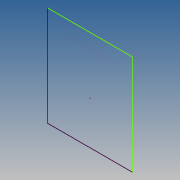
# Autodesk Inventor part: MountingBracket
Saved by Autodesk Inventor 2019 (Build 230136000, 136)
## iProperties
Created: 2019-12-19
Part Number: MountingBracket
Material: Generic
Document SubType Name: Modeling
Designer: voigt
Density: 1 g/cm^3
Appearance: Default
Author: voigt
Autodesk Inventor part; units mm, degrees
ref_plane "YZ Plane" through (0, 0, 0) normal (1, 0, 0) x (0, 1, 0)
ref_plane "XZ Plane" through (0, 0, 0) normal (0, 1, 0) x (-1, 0, 0)
ref_plane "XY Plane" through (0, 0, 0) normal (0, 0, 1) x (1, 0, 0)
sketch "Sketch1" plane through (0, 0, 0) normal (0, 0, 1) x (1, 0, 0)
  line L0 (20.828, 60.2998) -> (-20.828, 60.2998) construction
  line L1 (-38.1, 60.2998) -> (-38.1, 136.4998) construction
  line L2 (-38.1, 136.4998) -> (-20.828, 136.4998) construction
  line L3 (38.1, 136.4998) -> (-38.1, 136.4998) construction
  line L4 (37.846, 60.2998) -> (37.846, 136.4998) construction
  line L5 (-20.828, 47.6808) -> (-38.1, 47.6808) construction
  line L6 (-38.1, 136.4998) -> (37.846, 136.4998)
  line L7 (37.846, 136.4998) -> (37.846, 225.3188)
  line L8 (37.846, 225.3188) -> (-38.1, 225.3188)
  line L9 (-38.1, 225.3188) -> (-38.1, 136.4998)
  point P0 (0, 0)
  constraints: 8 end point, 2 parallel, 1 horizontal, 1 perpendicular
extrude "Extrusion1" add sketch "Sketch1" along normal blind 8
sketch "Sketch2" plane through (0, 0, 0) normal (0, 0, -1) x (-1, 0, 0)
  line L0 (-37.846, 136.4998) -> (-37.846, 225.3188) projected
  line L1 (38.1, 225.3188) -> (38.1, 136.4998) projected
  line L2 (-37.846, 225.3188) -> (38.1, 225.3188)
  line L3 (38.1, 225.3188) -> (38.1, 215.3188)
  line L4 (38.1, 215.3188) -> (-37.846, 215.3188)
  line L5 (-37.846, 215.3188) -> (-37.846, 225.3188)
  point P0 (0, 0)
  dimension "d2" = 10
  constraints: 8 end point, 2 parallel, 1 horizontal, 1 perpendicular, 1 point on line
  measures "d2" distance of L2.end L3.end
extrude "Extrusion2" add sketch "Sketch2" along normal blind 38
body "Solid1"
